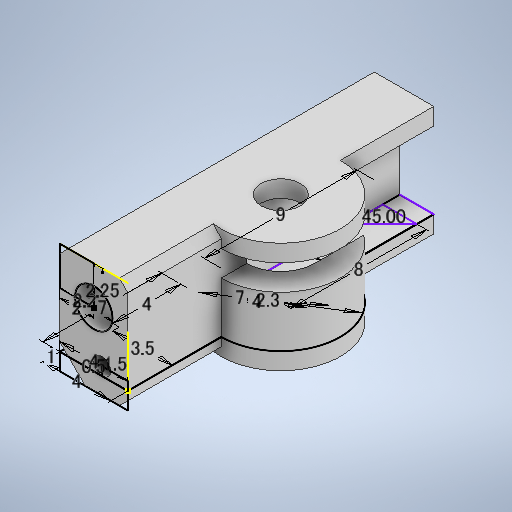
# Autodesk Inventor part: rod6.1
Saved by Autodesk Inventor 2025 (Build 290162000, 162)
## iProperties
Created: 2024-08-07
Part Number: rod6.1
Material: 一般
Document SubType Name: Modeling
Designer: Saigusa
Density: 1 g/cm^3
Appearance: 既定
Author: Saigusa
Autodesk Inventor part; units mm, degrees
ref_plane "YZ Plane" through (0, 0, 0) normal (1, 0, 0) x (0, 1, 0)
ref_plane "XZ Plane" through (0, 0, 0) normal (0, 1, 0) x (-1, 0, 0)
ref_plane "XY Plane" through (0, 0, 0) normal (0, 0, 1) x (1, 0, 0)
sketch "スケッチ1" plane through (0, 0, 0) normal (0, 1, 0) x (-1, 0, 0)
  circle A0 centre (0, 0) radius 1.15
  circle A1 centre (0, 0) radius 2
  circle A2 centre (0, 0) radius 3.5
  line L0 (0, 0) -> (0, 3.5)
  line L1 (2, 0) -> (-2, 0)
  line L2 (2, 0) -> (2, -2.8723)
  line L3 (-2, 0) -> (-2, -2.8723)
  line L4 (0, 2) -> (3.5, 2)
  line L5 (3.5, 2) -> (3.5, 6)
  line L6 (3.5, 6) -> (0, 6)
  line L7 (0, 6) -> (0, 2)
  line L8 (0, 6) -> (3.5, 6)
  line L9 (3.5, 6) -> (3.5, 0)
  line L10 (3.5, 0) -> (0, 0)
  line L11 (0, 0) -> (0, 6)
  line L12 (0, 0) -> (0, -8)
  line L13 (0, 0) -> (3.5, 0)
  line L14 (3.5, 0) -> (3.5, -8)
  line L15 (3.5, -8) -> (0, -8)
  line L16 (0, -8) -> (0, 0)
  line L17 (2, -2.8723) -> (2, -8)
  line L18 (0, -8) -> (3.5, -4.5)
  line L19 (0, -8) -> (4.9497, -8) construction
  line L20 (0, 0) -> (3.5, 0)
  line L21 (3.5, 0) -> (3.5, -9)
  line L22 (3.5, -9) -> (0, -9)
  line L23 (0, -9) -> (0, 0)
  line L24 (0, 2) -> (4, 2)
  line L25 (4, 2) -> (4, 9)
  line L26 (4, 9) -> (0, 9)
  line L27 (0, 9) -> (0, 2)
  line L28 (0, 9) -> (4, 9)
  line L29 (4, 9) -> (4, -9)
  line L30 (4, -9) -> (0, -9)
  line L31 (0, -9) -> (0, 9)
  line L32 (0, 0) -> (2, 0)
  line L33 (2, 0) -> (2, -9)
  line L34 (2, -9) -> (0, -9)
  line L35 (0, -9) -> (0, 0)
  point P0 (2, -6)
  point P1 (0, -3.5)
  dimension "d0" = 2.3
  dimension "d1" = 4
  dimension "d2" = 7
  dimension "d3" = 3.5
  dimension "d4" = 4
  dimension "d5" = 8
  dimension "d6" = 45
  dimension "d40" = 9
  dimension "d41" = 4
  dimension "d42" = 7
  constraints: 72 end point, 14 parallel, 11 perpendicular, 8 horizontal, 7 point on circle, 4 point on line, 3 centre point, 3 coincident, 2 vertical, 1 equal length, 1 midpoint
  measures "d0" diameter of A0
  measures "d1" diameter of A1
  measures "d2" diameter of A2
  measures "d3" distance of L6.end L5.end
  measures "d4" distance of L5.end L4.end
  measures "d5" distance of L10.end L12.end
  measures "d6" angle of L19 L18
  measures "d40" distance of L20.end L21.end
  measures "d41" distance of L26.end L25.end
  measures "d42" distance of L25.end L24.end
extrude "押し出し1" add sketch "スケッチ1" along normal blind 3 contours A1 L3 A2 L0
extrude "押し出し2" add sketch "スケッチ1" along normal blind 4.5 contours L10 A2 L2 | A1 L4 A2 L10 | L0 A2 L4 | A2 L14 L18 L17 | A2 L4 L9 | L9 L24 L29 L30 L21 L14 | L7 L6 L5 L4 A2 | L18 L14 L15 L17 | L5 L6 L27 L26 L25 L24 | L15 L21 L22 L33
extrude "押し出し3" add sketch "スケッチ1" against normal blind 1 contours L1 A1 L12 A0 | A0 L0 A1 L1 | A0 L1 A1 L0 | L12 A1 L1 A0 | L2 A2 L12 A1 | L10 A2 L2 | A1 L4 A2 L10 | A1 L3 A2 L0 | L0 A2 L4 | L12 A2 L3 A1 | L17 L18 L12 A2 | A2 L14 L18 L17 | A2 L4 L9 | L9 L24 L29 L30 L21 L14 | L7 L6 L5 L4 A2 | L18 L14 L15 L17 | L17 L15 L18 | L5 L6 L27 L26 L25 L24 | L15 L33 L22 L23 | L15 L21 L22 L33
sketch "スケッチ4" plane through (0, 4.5, 0) normal (0, 1, 0) x (1, 0, 0)
  circle A0 centre (0, 0) radius 1.15
  circle A1 centre (0, 0) radius 2
  circle A2 centre (0, 0) radius 3.5
  line L0 (-4, 9) -> (-4, -9) projected
  line L1 (0, 0) -> (-4, 0)
  line L2 (-4, 0) -> (-4, -9)
  line L3 (-4, -9) -> (0, -9)
  line L4 (0, -9) -> (0, 0)
  line L5 (0, 0) -> (-4, 0)
  line L6 (-4, 0) -> (-4, 9)
  line L7 (-4, 9) -> (0, 9)
  line L8 (0, 9) -> (0, 0)
  point P0 (0, -3.5)
  point P1 (0, 3.5)
  dimension "d43" = 2.3
  dimension "d44" = 4
  dimension "d45" = 7
  dimension "d46" = 4
  dimension "d47" = 9
  constraints: 16 end point, 4 parallel, 3 centre point, 3 coincident, 2 horizontal, 2 perpendicular
  measures "d43" diameter of A0
  measures "d44" diameter of A1
  measures "d45" diameter of A2
  measures "d46" distance of L6.end L7.end
  measures "d47" distance of L5.end L6.end
extrude "押し出し6" add sketch "スケッチ4" along normal blind 1 contours A0 L8 A1 L4 | A0 L1 A1 L8 | L4 A1 L1 A0 | L8 A2 L4 A1 | A1 L1 A2 L8 | L4 A2 L1 A1 | A2 L1 L0 L7 L8 | L4 L3 L0 L1 A2
sketch "スケッチ5" plane through (-4, -1, 9) normal (0, 0, 1) x (1, 0, 0)
  line L0 (4, 0) -> (4, 4) projected
  line L1 (4, 0) -> (0, 0)
  line L2 (0, 0) -> (0, 1)
  line L3 (0, 1) -> (4, 1)
  line L4 (4, 1) -> (4, 0)
  line L5 (4, 1) -> (2.5, 1)
  line L6 (2.5, 1) -> (2.5, 1.5)
  line L7 (2.5, 1.5) -> (4, 1.5)
  line L8 (4, 1.5) -> (4, 1)
  line L9 (4, 6.5) -> (0, 6.5) projected
  line L10 (0, 6.5) -> (2, 6.5)
  line L11 (2, 6.5) -> (2, 4.25)
  line L12 (2, 4.25) -> (0, 4.25)
  line L13 (0, 4.25) -> (0, 6.5)
  circle A0 centre (2, 4.25) radius 1.1
  dimension "d50" = 4
  dimension "d51" = 1
  dimension "d52" = 1.5
  dimension "d53" = 0.5
  dimension "d54" = 2
  dimension "d55" = 2.25
  dimension "d56" = 2.2
  constraints: 24 end point, 6 parallel, 3 horizontal, 3 perpendicular, 1 centre point, 1 coincident
  measures "d50" distance of L2.end L3.end
  measures "d51" distance of L1.end L2.end
  measures "d52" distance of L6.end L7.end
  measures "d53" distance of L5.end L6.end
  measures "d54" distance of L11.end L12.end
  measures "d55" distance of L10.end L11.end
  measures "d56" diameter of A0
extrude "押し出し7" cut sketch "スケッチ5" against normal blind 7 contours A0 L12 L11 | L11 L12 A0
hole "穴2" at (-1.5, 0.5, 9) direction (0, 0, -1) diameter 1 end through all
chamfer "面取り1" distance 0.5 angle 45 3 edges at (0, -1, 6.25) (0, 5.5, 6.25) (-4, 5.5, 0)
chamfer "面取り2" distance 1.5 angle 45 1 edges at (-4, -1, 0)
